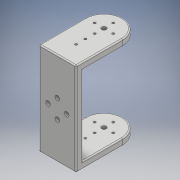
# Autodesk Inventor part: fork
Saved by Autodesk Inventor 2018 (Build 220112000, 112)
## iProperties
Created: 2018-04-07
Part Number: fork
Material: Generic
Document SubType Name: Modeling
Designer: Matyi
Density: 1 g/cm^3
Appearance: Default
Author: Matyi
Autodesk Inventor part; units mm, degrees
ref_plane "YZ Plane" through (0, 0, 0) normal (1, 0, 0) x (0, 1, 0)
ref_plane "XZ Plane" through (0, 0, 0) normal (0, 1, 0) x (-1, 0, 0)
ref_plane "XY Plane" through (0, 0, 0) normal (0, 0, 1) x (1, 0, 0)
sketch "Sketch11" plane through (0, 0, 0) normal (0, 1, 0) x (-1, 0, 0)
  line L0 (0, 0) -> (16, 0)
  line L1 (16, 0) -> (16, -40)
  line L2 (16, -40) -> (0, -40)
  line L3 (0, -40) -> (0, 0)
  circle A0 centre (8, -24) radius 1
  circle A1 centre (4, -20) radius 1
  circle A2 centre (8, -16) radius 1
  circle A3 centre (12, -20) radius 1
  dimension "d45" = 16
  dimension "d46" = 40
  dimension "d47" = 2
  dimension "d48" = 2
  dimension "d49" = 2
  dimension "d50" = 2
  dimension "d51" = 8
  dimension "d52" = 24
  dimension "d53" = 8
  dimension "d54" = 24
  dimension "d55" = 12
  dimension "d56" = 20
  dimension "d57" = 20
  dimension "d58" = 4
  constraints: 8 end point, 4 centre point, 2 parallel, 1 horizontal, 1 perpendicular
  measures "d45" distance of L1.end L2.end
  measures "d46" distance of L0.end L1.end
  measures "d47" diameter of A0
  measures "d48" diameter of A1
  measures "d49" diameter of A2
  measures "d50" diameter of A3
  measures "d51" distance from line of L1 A0.centre
  measures "d52" distance from line of L0 A0.centre
  measures "d53" distance from line of L3 A2.centre
  measures "d54" distance from line of L2 A2.centre
  measures "d55" distance from line of L1 A1.centre
  measures "d56" distance from line of L2 A1.centre
  measures "d57" distance from line of L2 A3.centre
  measures "d58" distance from line of L1 A3.centre
extrude "Extrusion6" add sketch "Sketch11" along normal blind 3
sketch "Sketch12" plane through (0, 3, 0) normal (0, 1, 0) x (1, 0, 0)
  line L0 (-16, 40) -> (-16, 0) projected
  line L1 (0, 0) -> (-16, 0)
  line L2 (-16, 0) -> (-16, 3)
  line L3 (-16, 3) -> (0, 3)
  line L4 (0, 3) -> (0, 0)
  line L5 (0, 40) -> (-16, 40)
  line L6 (-16, 40) -> (-16, 37)
  line L7 (-16, 37) -> (0, 37)
  line L8 (0, 37) -> (0, 40)
  dimension "d61" = 3
  dimension "d62" = 3
  constraints: 16 end point, 4 parallel, 3 point on line, 2 horizontal, 2 perpendicular
  measures "d61" distance of L1.end L2.end
  measures "d62" distance of L6.end L5.end
extrude "Extrusion7" add sketch "Sketch12" along normal blind 25
fillet "Fillet3" radius 8 4 edges at (0, 28, -1.5) (-16, 28, -1.5) (-16, 28, -38.5) (0, 28, -38.5)
sketch "Sketch13" plane through (-16, 0, 0) normal (0, 0, 1) x (1, 0, 0)
  circle A0 centre (8, 20) radius 1
  circle A1 centre (8, 16) radius 0.5
  line L0 (16, 0) -> (0, 0) projected
  line L1 (16, 0) -> (16, 20) projected
  circle A2 centre (8, 12) radius 0.5
  circle A3 centre (8, 24) radius 0.5
  circle A4 centre (12, 20) radius 0.5
  circle A5 centre (4, 20) radius 0.5
  circle A6 centre (8, 8) radius 0.5
  dimension "d66" = 2
  dimension "d67" = 1
  dimension "d68" = 20
  dimension "d69" = 8
  dimension "d70" = 8
  dimension "d71" = 16
  dimension "d72" = 1
  dimension "d73" = 1
  dimension "d74" = 1
  dimension "d75" = 1
  dimension "d76" = 1
  dimension "d77" = 4
  dimension "d78" = 8
  dimension "d79" = 4
  dimension "d80" = 20
  dimension "d81" = 4
  dimension "d82" = 20
  dimension "d83" = 8
  dimension "d84" = 8
  dimension "d85" = 8
  dimension "d86" = 12
  constraints: 7 centre point
  measures "d66" diameter of A0
  measures "d67" diameter of A1
  measures "d68" distance from line of L0 A0.centre
  measures "d69" distance from line of L1 A0.centre
  measures "d70" distance from line of L1 A1.centre
  measures "d71" distance from line of L0 A1.centre
  measures "d72" diameter of A2
  measures "d73" diameter of A3
  measures "d74" diameter of A4
  measures "d75" diameter of A5
  measures "d76" diameter of A6
  measures "d77" distance of A0.centre A3.centre
  measures "d78" distance from line of L1 A3.centre
  measures "d79" distance of A0.centre A4.centre
  measures "d80" distance from line of L0 A4.centre
  measures "d81" distance of A0.centre A5.centre
  measures "d82" distance from line of L0 A5.centre
  measures "d83" distance of A0.centre A2.centre
  measures "d84" distance from line of L1 A2.centre
  measures "d85" distance from line of L1 A6.centre
  measures "d86" distance of A0.centre A6.centre
sketch "Sketch14" plane through (0, 0, -40) normal (0, 0, -1) x (-1, 0, 0)
  circle A0 centre (8, 20) radius 1
  circle A1 centre (8, 16) radius 0.5
  circle A2 centre (8, 12) radius 0.5
  circle A3 centre (12, 20) radius 0.5
  circle A4 centre (8, 24) radius 0.5
  circle A5 centre (4, 20) radius 0.5
  circle A6 centre (8, 8) radius 0.5
  line L0 (16, 0) -> (16, 20) projected
  line L1 (16, 0) -> (0, 0) projected
  line L2 (0, 0) -> (0, 20) projected
  dimension "d87" = 2
  dimension "d88" = 1
  dimension "d89" = 1
  dimension "d90" = 1
  dimension "d91" = 1
  dimension "d92" = 1
  dimension "d93" = 1
  dimension "d94" = 8
  dimension "d95" = 20
  dimension "d96" = 20
  dimension "d97" = 4
  dimension "d98" = 4
  dimension "d99" = 8
  dimension "d100" = 4
  dimension "d101" = 20
  dimension "d102" = 4
  dimension "d103" = 8
  dimension "d104" = 8
  dimension "d105" = 8
  dimension "d106" = 12
  dimension "d107" = 8
  constraints: 7 centre point
  measures "d87" diameter of A0
  measures "d88" diameter of A1
  measures "d89" diameter of A2
  measures "d90" diameter of A3
  measures "d91" diameter of A4
  measures "d92" diameter of A5
  measures "d93" diameter of A6
  measures "d94" distance from line of L0 A0.centre
  measures "d95" distance from line of L1 A0.centre
  measures "d96" distance from line of L1 A3.centre
  measures "d97" distance of A0.centre A3.centre
  measures "d98" distance of A0.centre A4.centre
  measures "d99" distance from line of L2 A4.centre
  measures "d100" distance of A5.centre A0.centre
  measures "d101" distance from line of L1 A5.centre
  measures "d102" distance of A0.centre A1.centre
  measures "d103" distance from line of L0 A1.centre
  measures "d104" distance from line of L0 A2.centre
  measures "d105" distance of A0.centre A2.centre
  measures "d106" distance of A0.centre A6.centre
  measures "d107" distance from line of L0 A6.centre
extrude "Extrusion8" cut sketch "Sketch14" against normal blind 3
extrude "Extrusion9" cut sketch "Sketch13" against normal blind 3
fillet "Fillet4" radius 0.5 18 edges at (-16, 11.5003, -3) (0, 11.5003, -3) (-2.343, 25.657, -3) (0, 10.0003, 0) (-16, 10.0003, 0) (-2.343, 25.657, 0) (0, 3, -20) (0, 0, -20) (-16, 3, -20) (-13.657, 25.657, -37) (-16, 11.5003, -37) (0, 11.5003, -37) (-13.657, 25.657, -40) (-16, 10.0003, -40) (0, 10.0003, -40) (-8, 0, 0) (-16, 0, -20) (-8, 0, -40)
equation "\"d51\" = 0.5 * d45"
equation "\"d53\" = 0.5 * d45"
equation "\"d56\" = 0.5 * d46"
equation "\"d57\" = 0.5 * d46"
body "Solid2"
